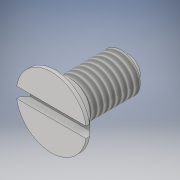
# Autodesk Inventor part: M8x16
Saved by Autodesk Inventor 2019.3 (Build 233278000, 278)
## iProperties
Created: 2020-04-01
Part Number: M8x16
Material: Типовые
Document SubType Name: Modeling
Designer: Admin
Density: 1 g/cm^3
Appearance: По умолчанию
Author: Admin
Autodesk Inventor part; units mm, degrees
ref_plane "YZ Plane" through (0, 0, 0) normal (1, 0, 0) x (0, 1, 0)
ref_plane "XZ Plane" through (0, 0, 0) normal (0, 1, 0) x (-1, 0, 0)
ref_plane "XY Plane" through (0, 0, 0) normal (0, 0, 1) x (1, 0, 0)
sketch "Эскиз1" plane through (0, 0, 0) normal (1, 0, 0) x (0, 1, 0)
  line L0 (7.25, 0) -> (7.25, -0.75)
  line L1 (7.25, -0.75) -> (4, -4)
  line L2 (4, -4) -> (4, -16)
  line L3 (7.25, 0) -> (0, 0)
  line L4 (4, -16) -> (0, -16)
  line L5 (0, 0) -> (0, -16)
  line L6 (0, -19.2) -> (0, 3.2) projected
  dimension "d7" = 8
  dimension "d8" = 14.5
  dimension "d9" = 4
  dimension "d10" = 16
  dimension "d11" = 45
  constraints: 12 end point, 1 horizontal, 1 vertical
  measures "d7" diameter of L5 L2
  measures "d8" diameter of L5 L0
  measures "d9" distance from line of L3 L1.end
  measures "d10" distance between parallel lines of L4 L3
  measures "d11" angle of L2 L1
revolve "Вращение1" add sketch "Эскиз1" angle 360 about axis through (0, 0, -10) along (0, 0, 1)
thread "Резьба1" size "M8x1.25" class "6g" standard "ANSI Metric M Profile" length 12
chamfer "Фаска1" distance 1.6 angle 45 1 edges at (0, -4, -16)
sketch "Эскиз2" plane through (0, 0, 0) normal (1, 0, 0) x (0, 1, 0)
  line L0 (1.1, 0) -> (1.1, -1.8)
  line L1 (1.1, -1.8) -> (-1.1, -1.8)
  line L2 (-1.1, -1.8) -> (-1.1, 0)
  line L3 (-1.1, 0) -> (1.1, 0)
  line L4 (0, -19.9863) -> (0, 7.9179) projected
  line L5 (-7.25, 0) -> (7.25, 0) projected
  point P0 (0, 0)
  dimension "d18" = 1.8
  dimension "d19" = 2.2
  constraints: 8 end point, 3 perpendicular, 1 point on line, 1 vertical, 1 other
  measures "d18" distance of L0.start L0.end
  measures "d19" distance of L2.end L0.start
extrude "Выдавливание1" cut sketch "Эскиз2" along normal through all both and the other way through all
